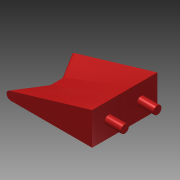
# Autodesk Inventor part: Bottom Pivot Mk1
Saved by Autodesk Inventor 2015 (Build 190159000, 159)
## iProperties
Created: 2016-11-23
Part Number: Bottom Pivot Mk1
Material: Generic
Document SubType Name: Modeling
Designer: Markus
Density: 1 g/cm^3
Appearance: Light Red
Author: Markus
Autodesk Inventor part; units mm, degrees
ref_plane "YZ Plane" through (0, 0, 0) normal (1, 0, 0) x (0, 1, 0)
sketch "Sketch1" plane through (0, 0, 0) normal (0, 0, 1) x (1, 0, 0)
  line L0 (0, 0) -> (0, 12.7)
  line L1 (0, 12.7) -> (-25.952, 3.0759)
  line L2 (0, 0) -> (-25.4, 0)
  arc A0 (-25.952, 3.0759) -> (-25.4, 0) centre (-25.4, 1.5875) ccw
  dimension "d0" = 25.4
  dimension "d1" = 3.175
  dimension "d2" = 12.7
  constraints: 6 end point, 2 point on circle, 2 tangent, 1 centre point, 1 horizontal, 1 vertical, 1 vertical alignment
  measures "d0" distance of L0.start L2.end
  measures "d1" diameter of A0
  measures "d2" distance of L0.start L0.end
extrude "Extrusion1" add sketch "Sketch1" along normal mid plane 5.08
ref_plane "Work Plane1" through (0, 0, 12.7) normal (0, 0, 1) x (1, 0, 0)
sketch "Sketch2" plane through (0, 0, 12.7) normal (0, 0, 1) x (1, 0, 0)
  arc A0 (-32.2031, 3.109) -> (-31.75, 0) centre (-31.75, 1.5875) ccw
  line L0 (0, 0) -> (-31.75, 0)
  line L1 (0, 0) -> (0, 12.7)
  line L2 (0, 12.7) -> (-32.2031, 3.109)
  line L3 (0, 12.7) -> (-25.952, 3.0759) construction
  dimension "d6" = 3.175
  dimension "d7" = 31.75
  constraints: 6 end point, 2 point on circle, 2 tangent, 1 centre point, 1 horizontal, 1 vertical, 1 vertical alignment
  measures "d6" diameter of A0
  measures "d7" distance of L0.start L0.end
ref_plane "Work Plane2" through (0, 0, -12.7) normal (0, 0, -1) x (-1, 0, 0)
sketch "Sketch3" plane through (0, 0, -12.7) normal (0, 0, -1) x (-1, 0, 0)
  line L0 (0, 12.7) -> (32.2031, 3.109) projected
  arc A0 (31.75, 0) -> (32.2031, 3.109) centre (31.75, 1.5875) ccw projected
  line L1 (0, 0) -> (31.75, 0) projected
  line L2 (0, 0) -> (0, 12.7) projected
loft "Loft1" add profiles "Sketch2" section 1 edges at (0, 6.35, 2.54) (-12.976, 7.888, 2.54) (-26.9625, 1.3071, 2.54) (-12.7, 0, 2.54)
loft "Loft2" add profiles "Sketch3" section 1 edges at (0, 6.35, -2.54) (-12.7, 0, -2.54) (-26.9625, 1.3071, -2.54) (-12.976, 7.888, -2.54)
sketch "Sketch4" plane through (0, 0, 12.7) normal (1, 0, 0) x (0, 0, -1)
  line L0 (15.24, 12.7) -> (10.16, 12.7) construction
  line L1 (10.16, 12.7) -> (0, 12.7) construction
  line L2 (0, 12.7) -> (0, 0) construction
  line L3 (0, 0) -> (25.4, 0) construction
  line L4 (25.4, 0) -> (25.4, 12.7) construction
  line L5 (15.24, 12.7) -> (25.4, 12.7) construction
  line L6 (0, 12.7) -> (12.7, 0) construction
  line L7 (12.7, 0) -> (25.4, 12.7) construction
  circle A0 centre (6.35, 6.35) radius 1.5875
  circle A1 centre (19.05, 6.35) radius 1.5875
  dimension "d17" = 3.175
  dimension "d18" = 3.175
  constraints: 4 end point, 2 centre point, 2 midpoint, 1 perpendicular
  measures "d17" diameter of A0
  measures "d18" diameter of A1
extrude "Extrusion2" add sketch "Sketch4" along normal blind 6.35
body "Solid1"
